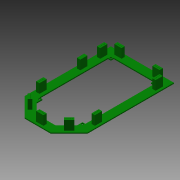
# Autodesk Inventor part: I2C
Saved by Autodesk Inventor 2015 (Build 190159000, 159)
## iProperties
Created: 2015-02-08
Part Number: I2C
Material: Generic
Document SubType Name: Modeling
Designer: Rafi Kurnia Putra
Density: 1 g/cm^3
Appearance: Dark Green
Mass: 24.0721 g
Surface Area: 249.214 cm^2
Volume: 24.0721 cm^3
Author: Rafi Kurnia Putra
Autodesk Inventor part; units mm, degrees
ref_plane "YZ Plane" through (0, 0, 0) normal (1, 0, 0) x (0, 1, 0)
ref_plane "XZ Plane" through (0, 0, 0) normal (0, 1, 0) x (-1, 0, 0)
ref_plane "XY Plane" through (0, 0, 0) normal (0, 0, 1) x (1, 0, 0)
sketch "Sketch1" plane through (0, 0, 0) normal (0, 1, 0) x (-1, 0, 0)
  line L0 (-27.8183, 73.3599) -> (-31.8913, 77.4328)
  line L1 (-32.6161, 71.4472) -> (-33.0686, 71.8997)
  line L2 (-31.7251, 73.2432) -> (-31.2726, 72.7907)
  line L3 (-31.9797, 73.2432) -> (-31.2726, 72.5361)
  line L4 (-31.2726, 73.6958) -> (-31.7251, 73.2432)
  line L5 (-31.2726, 72.7907) -> (-31.2726, 73.6958) construction
  line L6 (-31.2726, 72.7907) -> (-30.82, 73.2432)
  line L7 (-30.82, 73.2432) -> (-31.7251, 73.2432) construction
  line L8 (-31.2726, 73.9503) -> (-31.9797, 73.2432)
  line L9 (-31.2726, 72.5361) -> (-31.2726, 73.9503) construction
  line L10 (-30.82, 73.2432) -> (-31.2726, 73.6958)
  line L11 (-31.2726, 72.5361) -> (-30.5654, 73.2432)
  line L12 (-30.5654, 73.2432) -> (-31.9797, 73.2432) construction
  line L13 (-36.6607, 68.3076) -> (-37.1133, 67.8551)
  line L14 (-36.6607, 66.059) -> (-38.4568, 67.8551)
  line L15 (-37.1133, 67.8551) -> (-36.6607, 67.4025)
  line L16 (-40.8503, 68.4738) -> (-36.7774, 64.4008)
  line L17 (-36.6607, 67.4025) -> (-36.6607, 68.3076) construction
  line L18 (-47.7157, 32.4527) -> (-47.7157, 33.0927)
  line L19 (-47.7157, 33.0927) -> (-48.3557, 33.0927)
  line L20 (-48.3557, 33.0927) -> (-48.3557, 32.4527)
  line L21 (-48.3557, 32.4527) -> (-47.7157, 32.4527)
  line L22 (-47.7157, 32.4527) -> (-48.3557, 33.0927) construction
  line L23 (-47.7157, 33.0927) -> (-48.3557, 32.4527) construction
  circle A0 centre (-48.0357, 32.7727) radius 0.5
  line L24 (-46.7657, 31.5027) -> (-49.3057, 31.5027)
  line L25 (-48.3557, 35.6327) -> (-47.7157, 35.6327)
  line L26 (-46.7657, 41.6627) -> (-46.7657, 31.5027)
  line L27 (-49.3057, 31.5027) -> (-49.3057, 41.6627)
  line L28 (-45.6757, 30.2477) -> (-45.6757, 42.9177)
  line L29 (-51.4357, 42.9177) -> (-51.4357, 30.2477)
  line L30 (-48.3557, 34.9927) -> (-48.3557, 35.6327)
  line L31 (-48.3557, 34.9927) -> (-47.7157, 35.6327) construction
  line L32 (-47.7157, 35.6327) -> (-47.7157, 34.9927)
  line L33 (-47.7157, 34.9927) -> (-48.3557, 34.9927)
  circle A1 centre (-48.0357, 35.3127) radius 0.5
  line L34 (-51.4357, 30.2477) -> (-45.6757, 30.2477)
  line L35 (-48.3557, 35.6327) -> (-47.7157, 34.9927) construction
  line L36 (-48.3557, 37.5327) -> (-47.7157, 37.5327)
  circle A2 centre (-48.0357, 37.8527) radius 0.5
  line L37 (-47.7157, 38.1727) -> (-48.3557, 37.5327) construction
  line L38 (-47.7157, 37.5327) -> (-47.7157, 38.1727)
  line L39 (-47.7157, 37.5327) -> (-48.3557, 38.1727) construction
  line L40 (-47.7157, 38.1727) -> (-48.3557, 38.1727)
  line L41 (-48.3557, 38.1727) -> (-48.3557, 37.5327)
  line L42 (-48.3557, 40.0727) -> (-47.7157, 40.0727)
  line L43 (-48.3557, 40.7127) -> (-48.3557, 40.0727)
  line L44 (-47.7157, 40.0727) -> (-48.3557, 40.7127) construction
  line L45 (-47.7157, 40.7127) -> (-48.3557, 40.7127)
  line L46 (-47.7157, 40.0727) -> (-47.7157, 40.7127)
  line L47 (-47.7157, 40.7127) -> (-48.3557, 40.0727) construction
  line L48 (-47.5357, 39.8927) -> (-47.5357, 40.8927)
  line L49 (-48.5357, 40.8927) -> (-48.5357, 39.8927)
  line L50 (-47.5357, 40.8927) -> (-48.5357, 39.8927) construction
  line L51 (-47.5357, 39.8927) -> (-48.5357, 40.8927) construction
  line L52 (-47.5357, 40.8927) -> (-48.5357, 40.8927)
  line L53 (-48.5357, 39.8927) -> (-47.5357, 39.8927)
  line L54 (-49.3057, 41.6627) -> (-46.7657, 41.6627)
  line L55 (-45.6757, 42.9177) -> (-51.4357, 42.9177)
  line L56 (-22.8672, 91.7885) -> (-55.206, 59.4497)
  line L57 (-40.093, 53.1897) -> (-16.6072, 76.6755)
  line L58 (-33.0686, 70.9946) -> (-32.6161, 71.4472)
  line L59 (-36.2082, 67.8551) -> (-36.6607, 68.3076)
  line L60 (-36.2082, 67.8551) -> (-37.1133, 67.8551) construction
  line L61 (-36.6607, 67.4025) -> (-36.2082, 67.8551)
  circle A3 centre (-36.6607, 67.8551) radius 0.5
  line L62 (-34.8647, 69.1986) -> (-35.3172, 69.6511)
  line L63 (-35.3172, 69.6511) -> (-34.8647, 70.1037)
  line L64 (-34.8647, 70.1037) -> (-34.8647, 69.1986) construction
  line L65 (-34.4121, 69.6511) -> (-34.8647, 69.1986)
  line L66 (-35.3172, 69.6511) -> (-34.4121, 69.6511) construction
  line L67 (-34.8647, 70.1037) -> (-34.4121, 69.6511)
  circle A4 centre (-34.8647, 69.6511) radius 0.5
  line L68 (-31.8913, 77.4328) -> (-40.8503, 68.4738)
  line L69 (-38.4568, 67.8551) -> (-31.2726, 75.0393)
  line L70 (-36.7774, 64.4008) -> (-27.8183, 73.3599)
  line L71 (-29.4765, 73.2432) -> (-36.6607, 66.059)
  line L72 (-33.5212, 71.4472) -> (-33.0686, 70.9946)
  line L73 (-33.0686, 70.9946) -> (-33.0686, 71.8997) construction
  line L74 (-32.6161, 71.4472) -> (-33.5212, 71.4472) construction
  circle A5 centre (-33.0686, 71.4472) radius 0.5
  line L75 (-33.0686, 71.8997) -> (-33.5212, 71.4472)
  line L76 (-30.5654, 73.2432) -> (-31.2726, 73.9503)
  line L77 (-31.2726, 75.0393) -> (-29.4765, 73.2432)
  line L78 (40.093, 53.1893) -> (40.093, -76.6755)
  line L79 (40.093, -76.6755) -> (40.093, 53.1897)
  line L80 (55.206, -91.7885) -> (55.206, 59.4497)
  line L81 (55.206, 59.4497) -> (55.206, -91.7885)
  line L82 (-40.093, -76.6755) -> (-40.093, 53.1897)
  line L83 (-55.206, 59.4497) -> (-55.206, -91.7885)
  line L84 (45.676, -63.5823) -> (51.436, -63.5823)
  line L85 (47.536, -65.6073) -> (48.536, -65.6073)
  line L86 (47.536, -66.6073) -> (47.536, -65.6073)
  line L87 (47.536, -65.6073) -> (48.536, -66.6073) construction
  circle A6 centre (48.036, -73.7273) radius 0.5
  line L88 (46.766, -64.8373) -> (46.766, -74.9973)
  line L89 (11.7298, -91.7885) -> (54.9398, -91.7885)
  line L90 (40.093, -76.6755) -> (-40.093, -76.6755)
  line L91 (-55.206, -91.7885) -> (55.206, -91.7885)
  line L92 (49.306, -64.8373) -> (46.766, -64.8373)
  circle A7 centre (48.0357, 32.7727) radius 0.5
  line L93 (46.766, -74.9973) -> (49.306, -74.9973)
  line L94 (47.716, -68.3273) -> (48.356, -68.3273)
  line L95 (48.356, -68.9673) -> (47.716, -68.9673)
  line L96 (47.716, -68.3273) -> (48.356, -68.9673) construction
  line L97 (48.356, -68.3273) -> (48.356, -68.9673)
  line L98 (47.716, -68.9673) -> (48.356, -68.3273) construction
  circle A8 centre (48.036, -68.6473) radius 0.5
  line L99 (49.306, -74.9973) -> (49.306, -64.8373)
  line L100 (51.436, -63.5823) -> (51.436, -76.2523)
  line L101 (47.716, -73.4073) -> (48.356, -73.4073)
  line L102 (48.356, -73.4073) -> (48.356, -74.0473)
  line L103 (48.356, -74.0473) -> (47.716, -74.0473)
  line L104 (47.716, -73.4073) -> (48.356, -74.0473) construction
  line L105 (47.716, -74.0473) -> (48.356, -73.4073) construction
  line L106 (45.676, -76.2523) -> (45.676, -63.5823)
  line L107 (48.356, -65.7873) -> (48.356, -66.4273)
  line L108 (48.536, -66.6073) -> (47.536, -66.6073)
  line L109 (48.356, -66.4273) -> (47.716, -66.4273)
  line L110 (47.716, -66.4273) -> (47.716, -65.7873)
  line L111 (47.716, -65.7873) -> (48.356, -66.4273) construction
  line L112 (47.716, -65.7873) -> (48.356, -65.7873)
  line L113 (47.716, -66.4273) -> (48.356, -65.7873) construction
  line L114 (47.536, -66.6073) -> (48.536, -65.6073) construction
  line L115 (48.536, -65.6073) -> (48.536, -66.6073)
  line L116 (47.716, -68.9673) -> (47.716, -68.3273)
  line L117 (48.356, -70.8673) -> (47.716, -70.8673)
  line L118 (48.356, -71.5073) -> (48.356, -70.8673)
  line L119 (48.356, -70.8673) -> (47.716, -71.5073) construction
  line L120 (48.356, -71.5073) -> (47.716, -70.8673) construction
  line L121 (47.716, -71.5073) -> (48.356, -71.5073)
  line L122 (47.716, -70.8673) -> (47.716, -71.5073)
  circle A9 centre (48.036, -71.1873) radius 0.5
  line L123 (32.3848, -84.9385) -> (32.3848, -84.2985)
  line L124 (31.7448, -84.9385) -> (32.3848, -84.9385)
  line L125 (32.3848, -84.9385) -> (31.7448, -84.2985) construction
  line L126 (32.3848, -84.2985) -> (31.7448, -84.2985)
  line L127 (31.7448, -84.2985) -> (31.7448, -84.9385)
  line L128 (31.7448, -84.9385) -> (32.3848, -84.2985) construction
  circle A10 centre (29.5248, -84.6185) radius 0.5
  line L129 (28.2548, -83.3485) -> (28.2548, -85.8885)
  line L130 (26.9998, -88.0185) -> (26.9998, -82.2585)
  line L131 (38.4148, -85.8885) -> (38.4148, -83.3485)
  line L132 (29.8448, -84.2985) -> (29.8448, -84.9385)
  line L133 (29.2048, -84.2985) -> (29.8448, -84.2985)
  line L134 (29.8448, -84.2985) -> (29.2048, -84.9385) construction
  line L135 (29.2048, -84.9385) -> (29.2048, -84.2985)
  line L136 (29.2048, -84.2985) -> (29.8448, -84.9385) construction
  line L137 (29.8448, -84.9385) -> (29.2048, -84.9385)
  line L138 (34.9248, -84.2985) -> (34.9248, -84.9385)
  line L139 (34.9248, -84.2985) -> (34.2848, -84.9385) construction
  line L140 (34.9248, -84.9385) -> (34.2848, -84.9385)
  line L141 (34.2848, -84.2985) -> (34.9248, -84.2985)
  line L142 (34.2848, -84.2985) -> (34.9248, -84.9385) construction
  line L143 (34.2848, -84.9385) -> (34.2848, -84.2985)
  circle A11 centre (34.6048, -84.6185) radius 0.5
  line L144 (38.4148, -83.3485) -> (28.2548, -83.3485)
  line L145 (26.9998, -82.2585) -> (39.6698, -82.2585)
  line L146 (39.6698, -88.0185) -> (26.9998, -88.0185)
  line L147 (28.2548, -85.8885) -> (38.4148, -85.8885)
  circle A12 centre (32.0648, -84.6185) radius 0.5
  line L148 (47.716, -74.0473) -> (47.716, -73.4073)
  line L149 (39.6698, -82.2585) -> (39.6698, -88.0185)
  line L150 (51.436, -76.2523) -> (45.676, -76.2523)
  line L151 (-5.08, 85.8885) -> (-5.08, 83.3485)
  line L152 (-6.335, 82.2585) -> (-6.335, 88.0185)
  line L153 (22.8668, 91.7885) -> (-22.8672, 91.7885)
  line L154 (-16.6072, 76.6755) -> (16.6068, 76.6755)
  line L155 (16.6072, 76.6755) -> (-16.6068, 76.6755)
  line L156 (5.08, 83.3485) -> (5.08, 85.8885)
  circle A13 centre (3.81, 84.6187) radius 0.5
  circle A14 centre (1.27, 84.6185) radius 0.5
  line L157 (6.335, 88.0185) -> (6.335, 82.2585)
  line L158 (6.335, 82.2585) -> (-6.335, 82.2585)
  line L159 (-6.335, 88.0185) -> (6.335, 88.0185)
  line L160 (-5.08, 83.3485) -> (5.08, 83.3485)
  line L161 (31.2726, 75.0393) -> (29.4765, 73.2432)
  line L162 (27.8183, 73.3599) -> (31.8913, 77.4328)
  line L163 (31.7251, 73.2432) -> (31.2726, 72.7907)
  line L164 (31.9797, 73.2432) -> (31.2726, 72.5361)
  line L165 (31.2726, 72.7907) -> (30.82, 73.2432)
  line L166 (30.82, 73.2432) -> (31.7251, 73.2432) construction
  line L167 (31.2726, 73.6958) -> (31.7251, 73.2432)
  line L168 (31.2726, 72.7907) -> (31.2726, 73.6958) construction
  line L169 (30.5654, 73.2432) -> (31.9797, 73.2432) construction
  line L170 (31.2726, 73.9503) -> (31.9797, 73.2432)
  line L171 (31.2726, 72.5361) -> (30.5654, 73.2432)
  line L172 (31.2726, 72.5361) -> (31.2726, 73.9503) construction
  line L173 (30.82, 73.2432) -> (31.2726, 73.6958)
  line L174 (30.5654, 73.2432) -> (31.2726, 73.9503)
  line L175 (33.0686, 71.8997) -> (33.5212, 71.4472)
  line L176 (33.5212, 71.4472) -> (33.0686, 70.9946)
  line L177 (32.6161, 71.4472) -> (33.5212, 71.4472) construction
  line L178 (33.0686, 70.9946) -> (33.0686, 71.8997) construction
  line L179 (32.6161, 71.4472) -> (33.0686, 71.8997)
  line L180 (33.0686, 70.9946) -> (32.6161, 71.4472)
  circle A15 centre (33.0686, 71.4472) radius 0.5
  line L181 (34.4121, 69.6511) -> (34.8647, 69.1986)
  line L182 (34.8647, 70.1037) -> (34.4121, 69.6511)
  line L183 (34.8647, 69.1986) -> (35.3172, 69.6511)
  line L184 (35.3172, 69.6511) -> (34.8647, 70.1037)
  line L185 (35.3172, 69.6511) -> (34.4121, 69.6511) construction
  circle A16 centre (34.8647, 69.6511) radius 0.5
  line L186 (29.4765, 73.2432) -> (36.6607, 66.059)
  line L187 (34.8647, 70.1037) -> (34.8647, 69.1986) construction
  line L188 (36.2082, 67.8551) -> (36.6607, 68.3076)
  line L189 (36.6607, 67.4025) -> (36.6607, 68.3076) construction
  line L190 (36.6607, 67.4025) -> (36.2082, 67.8551)
  line L191 (55.206, 59.4493) -> (22.8668, 91.7885)
  line L192 (16.6068, 76.6755) -> (40.093, 53.1893)
  line L193 (36.6607, 68.3076) -> (37.1133, 67.8551)
  line L194 (36.2082, 67.8551) -> (37.1133, 67.8551) construction
  circle A17 centre (36.6607, 67.8551) radius 0.5
  line L195 (40.093, 53.1897) -> (16.6072, 76.6755)
  line L196 (36.7774, 64.4008) -> (27.8183, 73.3599)
  line L197 (36.6607, 66.059) -> (38.4568, 67.8551)
  line L198 (38.4568, 67.8551) -> (31.2726, 75.0393)
  line L199 (31.8913, 77.4328) -> (40.8503, 68.4738)
  line L200 (22.8672, 91.7885) -> (55.206, 59.4497)
  line L201 (40.8503, 68.4738) -> (36.7774, 64.4008)
  line L202 (48.5357, 39.8927) -> (47.5357, 39.8927)
  line L203 (48.3557, 40.0727) -> (47.7157, 40.0727)
  line L204 (47.7157, 40.0727) -> (48.3557, 40.7127) construction
  line L205 (48.3557, 40.7127) -> (48.3557, 40.0727)
  line L206 (47.7157, 40.0727) -> (47.7157, 40.7127)
  line L207 (47.7157, 40.7127) -> (48.3557, 40.7127)
  line L208 (47.7157, 40.7127) -> (48.3557, 40.0727) construction
  line L209 (48.5357, 40.8927) -> (48.5357, 39.8927)
  line L210 (47.5357, 40.8927) -> (48.5357, 39.8927) construction
  line L211 (47.5357, 39.8927) -> (48.5357, 40.8927) construction
  line L212 (47.5357, 40.8927) -> (48.5357, 40.8927)
  line L213 (47.7157, 37.5327) -> (48.3557, 38.1727) construction
  line L214 (47.5357, 39.8927) -> (47.5357, 40.8927)
  line L215 (48.3557, 37.5327) -> (47.7157, 37.5327)
  line L216 (37.1133, 67.8551) -> (36.6607, 67.4025)
  line L217 (45.6757, 42.9177) -> (51.4357, 42.9177)
  line L218 (49.3057, 41.6627) -> (46.7657, 41.6627)
  line L219 (48.3557, 34.9927) -> (48.3557, 35.6327)
  line L220 (48.3557, 34.9927) -> (47.7157, 35.6327) construction
  line L221 (47.7157, 34.9927) -> (48.3557, 34.9927)
  line L222 (47.7157, 35.6327) -> (47.7157, 34.9927)
  circle A18 centre (48.0357, 35.3127) radius 0.5
  line L223 (48.3557, 35.6327) -> (47.7157, 35.6327)
  line L224 (48.3557, 33.0927) -> (48.3557, 32.4527)
  line L225 (48.3557, 32.4527) -> (47.7157, 32.4527)
  line L226 (47.7157, 32.4527) -> (48.3557, 33.0927) construction
  line L227 (47.7157, 33.0927) -> (48.3557, 33.0927)
  line L228 (47.7157, 32.4527) -> (47.7157, 33.0927)
  line L229 (47.7157, 33.0927) -> (48.3557, 32.4527) construction
  line L230 (46.7657, 31.5027) -> (49.3057, 31.5027)
  line L231 (51.4357, 30.2477) -> (45.6757, 30.2477)
  circle A19 centre (48.0357, 37.8527) radius 0.5
  line L232 (49.3057, 31.5027) -> (49.3057, 41.6627)
  line L233 (46.7657, 41.6627) -> (46.7657, 31.5027)
  line L234 (45.6757, 30.2477) -> (45.6757, 42.9177)
  line L235 (51.4357, 42.9177) -> (51.4357, 30.2477)
  line L236 (47.7157, 38.1727) -> (48.3557, 37.5327) construction
  line L237 (48.3557, 38.1727) -> (48.3557, 37.5327)
  line L238 (47.7157, 37.5327) -> (47.7157, 38.1727)
  line L239 (48.3557, 35.6327) -> (47.7157, 34.9927) construction
  line L240 (47.7157, 38.1727) -> (48.3557, 38.1727)
  line L241 (-47.716, -68.3273) -> (-48.356, -68.3273)
  line L242 (-47.716, -68.3273) -> (-48.356, -68.9673) construction
  line L243 (-47.716, -68.9673) -> (-48.356, -68.3273) construction
  line L244 (-48.356, -68.3273) -> (-48.356, -68.9673)
  line L245 (-48.356, -68.9673) -> (-47.716, -68.9673)
  circle A20 centre (-48.036, -68.6473) radius 0.5
  line L246 (-47.716, -68.9673) -> (-47.716, -68.3273)
  line L247 (-45.676, -63.5823) -> (-51.436, -63.5823)
  line L248 (-49.306, -64.8373) -> (-46.766, -64.8373)
  line L249 (-48.536, -66.6073) -> (-47.536, -66.6073)
  line L250 (-48.356, -66.4273) -> (-47.716, -66.4273)
  line L251 (-47.716, -65.7873) -> (-48.356, -65.7873)
  line L252 (-47.716, -66.4273) -> (-48.356, -65.7873) construction
  line L253 (-47.716, -66.4273) -> (-47.716, -65.7873)
  line L254 (-47.716, -65.7873) -> (-48.356, -66.4273) construction
  line L255 (-48.356, -65.7873) -> (-48.356, -66.4273)
  line L256 (-48.536, -65.6073) -> (-48.536, -66.6073)
  line L257 (-47.536, -66.6073) -> (-48.536, -65.6073) construction
  line L258 (-47.536, -66.6073) -> (-47.536, -65.6073)
  line L259 (-47.536, -65.6073) -> (-48.536, -66.6073) construction
  line L260 (-47.536, -65.6073) -> (-48.536, -65.6073)
  line L261 (-32.3848, -84.9385) -> (-32.3848, -84.2985)
  line L262 (-31.7448, -84.9385) -> (-32.3848, -84.9385)
  line L263 (-29.8448, -84.9385) -> (-29.2048, -84.9385)
  line L264 (-29.2048, -84.9385) -> (-29.2048, -84.2985)
  line L265 (-29.2048, -84.2985) -> (-29.8448, -84.9385) construction
  line L266 (-36.6448, -85.1185) -> (-36.6448, -84.1185)
  line L267 (-36.8248, -84.9385) -> (-36.8248, -84.2985)
  line L268 (-36.8248, -84.2985) -> (-37.4648, -84.9385) construction
  line L269 (-37.4648, -84.2985) -> (-36.8248, -84.9385) construction
  line L270 (-36.8248, -84.2985) -> (-37.4648, -84.2985)
  line L271 (-37.4648, -84.2985) -> (-37.4648, -84.9385)
  line L272 (-36.6448, -84.1185) -> (-37.6448, -84.1185)
  line L273 (-37.6448, -85.1185) -> (-36.6448, -85.1185)
  line L274 (-36.6448, -84.1185) -> (-37.6448, -85.1185) construction
  line L275 (-37.6448, -84.1185) -> (-37.6448, -85.1185)
  line L276 (-38.4148, -85.8885) -> (-38.4148, -83.3485)
  line L277 (-37.4648, -84.9385) -> (-36.8248, -84.9385)
  line L278 (-29.2048, -84.2985) -> (-29.8448, -84.2985)
  line L279 (-29.8448, -84.2985) -> (-29.8448, -84.9385)
  line L280 (-29.8448, -84.2985) -> (-29.2048, -84.9385) construction
  line L281 (-32.3848, -84.9385) -> (-31.7448, -84.2985) construction
  circle A21 centre (-32.0648, -84.6185) radius 0.5
  line L282 (-26.9998, -82.2585) -> (-39.6698, -82.2585)
  line L283 (-39.6698, -88.0185) -> (-26.9998, -88.0185)
  line L284 (-38.4148, -83.3485) -> (-28.2548, -83.3485)
  line L285 (-28.2548, -85.8885) -> (-38.4148, -85.8885)
  line L286 (-34.2848, -84.9385) -> (-34.2848, -84.2985)
  line L287 (-34.2848, -84.2985) -> (-34.9248, -84.2985)
  line L288 (-34.9248, -84.2985) -> (-34.2848, -84.9385) construction
  line L289 (-34.9248, -84.2985) -> (-34.9248, -84.9385)
  line L290 (-34.9248, -84.9385) -> (-34.2848, -84.9385)
  line L291 (-34.2848, -84.2985) -> (-34.9248, -84.9385) construction
  circle A22 centre (-34.6048, -84.6185) radius 0.5
  line L292 (-47.716, -71.5073) -> (-48.356, -71.5073)
  line L293 (-48.356, -71.5073) -> (-48.356, -70.8673)
  line L294 (-48.356, -70.8673) -> (-47.716, -70.8673)
  line L295 (-46.766, -64.8373) -> (-46.766, -74.9973)
  line L296 (-49.306, -74.9973) -> (-49.306, -64.8373)
  line L297 (-51.436, -63.5823) -> (-51.436, -76.2523)
  line L298 (-45.676, -76.2523) -> (-45.676, -63.5823)
  line L299 (-47.716, -70.8673) -> (-47.716, -71.5073)
  line L300 (-48.356, -70.8673) -> (-47.716, -71.5073) construction
  line L301 (-48.356, -71.5073) -> (-47.716, -70.8673) construction
  circle A23 centre (-48.036, -71.1873) radius 0.5
  line L302 (-47.716, -73.4073) -> (-48.356, -73.4073)
  line L303 (-47.716, -74.0473) -> (-47.716, -73.4073)
  line L304 (-48.356, -74.0473) -> (-47.716, -74.0473)
  line L305 (-47.716, -74.0473) -> (-48.356, -73.4073) construction
  line L306 (-48.356, -73.4073) -> (-48.356, -74.0473)
  line L307 (-47.716, -73.4073) -> (-48.356, -74.0473) construction
  circle A24 centre (-48.036, -73.7273) radius 0.5
  line L308 (-46.766, -74.9973) -> (-49.306, -74.9973)
  line L309 (-51.436, -76.2523) -> (-45.676, -76.2523)
  line L310 (-31.7448, -84.2985) -> (-31.7448, -84.9385)
  line L311 (-31.7448, -84.9385) -> (-32.3848, -84.2985) construction
  line L312 (-32.3848, -84.2985) -> (-31.7448, -84.2985)
  circle A25 centre (-29.5248, -84.6185) radius 0.5
  line L313 (-28.2548, -83.3485) -> (-28.2548, -85.8885)
  line L314 (-26.9998, -88.0185) -> (-26.9998, -82.2585)
  line L315 (-37.6448, -84.1185) -> (-36.6448, -85.1185) construction
  line L316 (-39.6698, -82.2585) -> (-39.6698, -88.0185)
  line L317 (36.6448, -85.1185) -> (36.6448, -84.1185)
  line L318 (36.8248, -84.9385) -> (36.8248, -84.2985)
  line L319 (37.4648, -84.9385) -> (36.8248, -84.9385)
  line L320 (36.8248, -84.2985) -> (37.4648, -84.9385) construction
  line L321 (37.4648, -84.2985) -> (37.4648, -84.9385)
  line L322 (37.4648, -84.2985) -> (36.8248, -84.9385) construction
  line L323 (37.6448, -84.1185) -> (36.6448, -85.1185) construction
  line L324 (37.6448, -84.1185) -> (37.6448, -85.1185)
  line L325 (37.6448, -85.1185) -> (36.6448, -85.1185)
  line L326 (36.6448, -84.1185) -> (37.6448, -85.1185) construction
  line L327 (36.6448, -84.1185) -> (37.6448, -84.1185)
  line L328 (36.8248, -84.2985) -> (37.4648, -84.2985)
  line L329 (5.08, 85.8885) -> (-5.08, 85.8885)
  circle A26 centre (-1.27, 84.6185) radius 0.5
  line L330 (-3.31, 84.1185) -> (-4.31, 84.1185)
  line L331 (-4.31, 84.1185) -> (-4.31, 85.1185)
  line L332 (-4.31, 85.1185) -> (-3.31, 85.1185)
  line L333 (-3.31, 85.1185) -> (-3.31, 84.1185)
  line L334 (-3.31, 84.1185) -> (-4.31, 85.1185) construction
  line L335 (-4.31, 84.1185) -> (-3.31, 85.1185) construction
  line L336 (4.13, 84.2987) -> (3.49, 84.2987)
  line L337 (3.49, 84.2987) -> (3.49, 84.9387)
  line L338 (3.49, 84.9387) -> (4.13, 84.9387)
  line L339 (4.13, 84.9387) -> (4.13, 84.2987)
  line L340 (4.13, 84.2987) -> (3.49, 84.9387) construction
  line L341 (3.49, 84.2987) -> (4.13, 84.9387) construction
  line L342 (1.5903, 84.2987) -> (0.9503, 84.2987)
  line L343 (0.9503, 84.2987) -> (0.9503, 84.9387)
  line L344 (0.9503, 84.9387) -> (1.5903, 84.9387)
  line L345 (1.5903, 84.9387) -> (1.5903, 84.2987)
  line L346 (1.5903, 84.2987) -> (0.9503, 84.9387) construction
  line L347 (0.9503, 84.2987) -> (1.5903, 84.9387) construction
  line L348 (-0.95, 84.2985) -> (-1.59, 84.2985)
  line L349 (-1.59, 84.2985) -> (-1.59, 84.9385)
  line L350 (-1.59, 84.9385) -> (-0.95, 84.9385)
  line L351 (-0.95, 84.9385) -> (-0.95, 84.2985)
  line L352 (-0.95, 84.2985) -> (-1.59, 84.9385) construction
  line L353 (-1.59, 84.2985) -> (-0.95, 84.9385) construction
  line L354 (-3.49, 84.2985) -> (-4.13, 84.2985)
  line L355 (-4.13, 84.2985) -> (-4.13, 84.9385)
  line L356 (-4.13, 84.9385) -> (-3.49, 84.9385)
  line L357 (-3.49, 84.9385) -> (-3.49, 84.2985)
  line L358 (-3.49, 84.2985) -> (-4.13, 84.9385) construction
  line L359 (-4.13, 84.2985) -> (-3.49, 84.9385) construction
  point P0 (-31.2726, 73.2432)
  point P1 (-31.2726, 73.2432)
  point P2 (-31.2726, 73.2432)
  point P3 (-48.0357, 40.3927)
  point P4 (-48.0357, 40.3927)
  point P5 (-48.0357, 40.3927)
  point P6 (-48.0357, 40.3927)
  point P7 (-31.2726, 73.2432)
  point P8 (48.036, -66.1073)
  point P9 (48.036, -66.1073)
  point P10 (48.036, -66.1073)
  point P11 (48.036, -66.1073)
  point P12 (31.2726, 73.2432)
  point P13 (31.2726, 73.2432)
  point P14 (31.2726, 73.2432)
  point P15 (31.2726, 73.2432)
  point P16 (48.0357, 40.3927)
  point P17 (48.0357, 40.3927)
  point P18 (48.0357, 40.3927)
  point P19 (48.0357, 40.3927)
  point P20 (-53.556, -61.1673)
  point P21 (-43.556, -61.1673)
  point P22 (-48.036, -66.1073)
  point P23 (-48.036, -66.1073)
  point P24 (-48.036, -66.1073)
  point P25 (-48.036, -66.1073)
  point P26 (-37.1448, -84.6185)
  point P27 (-37.1448, -84.6185)
  point P28 (-37.1448, -84.6185)
  point P29 (-37.1448, -84.6185)
  point P30 (-42.0848, -90.1385)
  point P31 (-42.0848, -80.1385)
  point P32 (37.1448, -84.6185)
  point P33 (37.1448, -84.6185)
  point P34 (37.1448, -84.6185)
  point P35 (37.1448, -84.6185)
  point P36 (1.27, 84.6185)
  point P37 (-3.81, 84.6185)
  point P38 (1.2703, 84.6187)
  dimension "d521" = 15.113
  dimension "d522" = 15.113
  dimension "d523" = 15.113
  dimension "d551" = 5.76
  dimension "d552" = 2.54
  dimension "d556" = 1
  dimension "d557" = 1
  dimension "d558" = 2.54
  dimension "d560" = 1.27
  dimension "d561" = 2.54
  dimension "d563" = 2.54
  dimension "d564" = 0.64
  dimension "d565" = 0.64
  dimension "d566" = 0.64
  dimension "d567" = 0.64
  dimension "d568" = 0.64
  dimension "d569" = 0.64
  dimension "d570" = 0.64
  dimension "d571" = 0.64
  constraints: 720 end point, 114 midpoint, 66 parallel, 33 perpendicular, 27 centre point, 8 horizontal, 3 point on line, 3 vertical, 2 other
  measures "d521" distance between parallel lines of L91 L90
  measures "d522" distance between parallel lines of L80 L78
  measures "d523" distance between parallel lines of L82 L83
  measures "d551" distance of L152.start L152.end
  measures "d552" distance of L151.start L151.end
  measures "d556" distance of L331.end L332.end
  measures "d557" distance of L330.end L331.end
  measures "d558" distance of A26.centre point (-3.81, 84.618)
  measures "d560" distance from line of A13.centre L156
  measures "d561" distance of point (1.27, 84.618) A13.centre
  measures "d563" distance of A26.centre point (1.27, 84.618)
  measures "d564" distance of L337.end L338.end
  measures "d565" distance of L336.end L337.end
  measures "d566" distance of L343.end L344.end
  measures "d567" distance of L342.end L343.end
  measures "d568" distance of L349.end L350.end
  measures "d569" distance of L348.end L349.end
  measures "d570" distance of L355.end L356.end
  measures "d571" distance of L354.end L355.end
extrude "Extrusion1" add sketch "Sketch1" along normal blind 1.7 contours L153 L191 L80 L91 L89 L83 L56
extrude "Extrusion2" add sketch "Sketch1" along normal blind 17.8 contours L70 L16 L68 L0 | L14 L69 L77 L71 | L24 L27 L54 L26 | L34 L29 L55 L28 | L84 L100 L150 L106 | L92 L99 L93 L88 | L144 L131 L147 L129 | L130 L145 L149 L146 | L329 L156 L160 L151 | L152 L159 L157 L158 | L198 L197 L186 L161 | L162 L199 L201 L196 | L217 L235 L231 L234 | L232 L230 L233 L218 | L298 L309 L297 L247 | L248 L295 L308 L296 | L276 L284 L313 L285 | L314 L283 L316 L282
sketch "Sketch2" plane through (0, 1.7, 0) normal (0, 1, 0) x (1, 0, 0)
  line L0 (-51.436, 63.5823) -> (-45.676, 63.5823) projected
  line L1 (-45.676, 63.5823) -> (-45.676, 76.2523) projected
  line L2 (-51.436, 76.2523) -> (-51.436, 63.5823) projected
  line L3 (-45.676, 76.2523) -> (-51.436, 76.2523) projected
  line L4 (-46.766, 39.9973) -> (-49.306, 39.9973)
  line L5 (-47.8892, 38.6529) -> (-47.8892, 38.0129)
  line L6 (-48.5292, 38.6529) -> (-47.8892, 38.6529)
  line L7 (-48.5292, 38.0129) -> (-47.8892, 38.6529) construction
  line L8 (-47.8892, 38.0129) -> (-48.5292, 38.0129)
  line L9 (-48.5292, 38.6529) -> (-47.8892, 38.0129) construction
  circle A0 centre (-48.2092, 38.3329) radius 0.5
  line L10 (-49.306, 39.9973) -> (-49.306, 29.8373)
  line L11 (-46.766, 29.8373) -> (-46.766, 39.9973)
  line L12 (-51.436, 28.5823) -> (-51.436, 41.2523)
  line L13 (-45.676, 41.2523) -> (-45.676, 28.5823)
  line L14 (-51.436, 41.2523) -> (-45.676, 41.2523)
  line L15 (-49.306, 29.8373) -> (-46.766, 29.8373)
  line L16 (-45.676, 28.5823) -> (-51.436, 28.5823)
  line L17 (-48.5292, 38.0129) -> (-48.5292, 38.6529)
  point P0 (0, 0)
  point P1 (-48.036, 29.8373)
  dimension "d578" = 1.09
  dimension "d579" = 22.33
  constraints: 28 end point, 3 midpoint, 1 centre point, 1 vertical alignment
  measures "d578" distance between parallel lines of L11 L13
  measures "d579" distance between parallel lines of L14 L0
extrude "Extrusion4" add sketch "Sketch2" along normal blind 16.1 contours L11 L15 L10 L4 | L5 L8 L17 L6 | A0 | L12 L14 L13 L16
sketch "Sketch4" plane through (0, 0, 0) normal (0, -1, 0) x (1, 0, 0)
  line L0 (-40.093, 53.1893) -> (-40.093, 48.1893)
  line L1 (-40.093, 48.1893) -> (-35.093, 48.1893)
  line L2 (-35.093, 48.1893) -> (-35.093, 58.1893)
  circle A0 centre (-37.593, 50.6893) radius 1.75
  line L3 (-40.093, -76.6755) -> (-35.093, -76.6755)
  line L4 (-35.093, -76.6755) -> (-35.093, -71.6755)
  line L5 (-35.093, -71.6755) -> (-40.093, -71.6755)
  line L6 (-40.093, -71.6755) -> (-40.093, -76.6755)
  circle A1 centre (-37.593, -74.1755) radius 1.75
  line L7 (40.093, 53.1897) -> (40.093, 48.1893)
  line L8 (40.093, 48.1893) -> (35.093, 48.1893)
  line L9 (35.093, 48.1893) -> (35.093, 58.1897)
  circle A2 centre (37.593, 50.6893) radius 1.75
  line L10 (40.093, -76.6755) -> (35.093, -76.6755)
  line L11 (35.093, -76.6755) -> (35.093, -71.6755)
  line L12 (35.093, -71.6755) -> (40.093, -71.6755)
  line L13 (40.093, -71.6755) -> (40.093, -76.6755)
  circle A3 centre (37.593, -74.1755) radius 1.75
  line L14 (-40.093, 53.1893) -> (-35.093, 58.1893)
  line L15 (35.093, 58.1897) -> (40.093, 53.1897)
  point P0 (0, 0)
  dimension "d596" = 5
  dimension "d597" = 5
  dimension "d599" = 5
  dimension "d600" = 5
  dimension "d602" = 10
  dimension "d603" = 7.0711
  dimension "d604" = 3.5
  dimension "d605" = 2.5
  dimension "d606" = 2.5
  dimension "d609" = 3.5
  dimension "d610" = 2.5
  dimension "d611" = 2.5
  constraints: 32 end point, 4 centre point, 3 perpendicular, 2 parallel, 1 horizontal
  measures "d596" distance of L0.start L0.end
  measures "d597" distance of L0.end L1.end
  measures "d599" distance of L5.end L4.end
  measures "d600" distance of L4.end L3.end
  measures "d602" distance of L1.end L2.end
  measures "d603" distance of L0.start L2.end
  measures "d604" diameter of A0
  measures "d605" distance from line of L2 A0.centre
  measures "d606" distance from line of L1 A0.centre
  measures "d609" diameter of A1
  measures "d610" distance from line of A1.centre L4
  measures "d611" distance from line of L5 A1.centre
extrude "Extrusion6" add sketch "Sketch4" against normal blind 1.7
body "Solid1"
